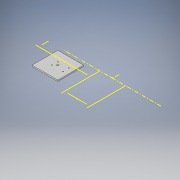
# Autodesk Inventor part: BT002_trajan20_21
Saved by Autodesk Inventor 2022.2 (Build 262287000, 287)
## iProperties
Company: HTBLA Kaindorf
RuleStatus: InUse
Created: 2022-06-07
Part Number: BT002_trajan20_21
Project: Zeichenmaschine_v2
Material: Generisch
Description: GM_Platte
Document SubType Name: Modeling
Designer: trajan20
Density: 1 g/cm^3
Appearance: Vorgabe
Mass: 25.3953 g
Surface Area: 141.888 cm^2
Volume: 25.3953 cm^3
AfterDocNew0: iProperties-Editor_aufrufen
Author: jan
Keywords: 2021
Autodesk Inventor part; units mm, degrees
ref_plane "YZ Plane" through (0, 0, 0) normal (1, 0, 0) x (0, 1, 0)
ref_plane "XZ Plane" through (0, 0, 0) normal (0, 1, 0) x (-1, 0, 0)
ref_plane "XY Plane" through (0, 0, 0) normal (0, 0, 1) x (1, 0, 0)
derived "MS000_trajan20_21_Zeichenmaschine_Inventor_Masterskizze.ipt"
sketch "Skizze19" plane through (30, -140, -50) normal (1, 0, 0) x (0, 1, 0)
  line L0 (10, -4) -> (-70, -4)
  line L1 (-70, -4) -> (-70, 0)
  line L2 (-70, 0) -> (10, 0)
  line L3 (10, 0) -> (10, -4)
  line L4 (-50, 10) -> (-10, 10)
  point P0 (140, 50)
  point P1 (-60, 0)
  point P2 (0, 0)
sketch "Basis" plane through (0, 0, 0) normal (0, 0, 1) x (1, 0, 0)
  line L0 (0, 150) -> (0, -150)
  line L1 (-19.8908, 0) -> (0.1065, 0)
  line L2 (0, -9.9039) -> (0, 9.9039)
  line L3 (30, -50) -> (30, -210)
  line L4 (0, -200) -> (20, -200)
  line L5 (0, -40) -> (120, -40)
  line L6 (0, 40) -> (120, 40)
  line L7 (110, -30) -> (110, 30)
  point P0 (0, 0)
  point P1 (110, 0)
sketch "Skizze20" plane through (30, -210, -54) normal (0, 0, 1) x (1, 0, 0)
  line L0 (0, 80) -> (0, 0)
  line L1 (0, 40) -> (-76.2792, 40) construction
  line L2 (-30, -72) -> (-30, 432) construction
  line L3 (-39.185, 86.341) -> (-39.185, 32.94) construction
  line L4 (-20.815, 77.6067) -> (-20.815, 18.0773) construction
  line L5 (-55.3723, 65.32) -> (-12.0627, 65.32) construction
  line L6 (-51.5852, 30.95) -> (-17.9084, 30.95) construction
  circle A0 centre (-30, 40) radius 3
  circle A1 centre (-20.815, 30.95) radius 1.35
  circle A2 centre (-39.185, 30.95) radius 1.35
  circle A3 centre (-39.185, 65.32) radius 1.35
  circle A4 centre (-20.815, 65.32) radius 1.35
  point P0 (-30, 210)
extrude "Extrusion3" add sketch "Skizze19" along normal blind 10 and the other way blind 30
mirror "Spiegeln1" about plane through (0, -170, -52) normal (-1, 0, 0)
extrude "Extrusion4" cut sketch "Skizze20" along normal through all
equation "\"d5\" = 0.5 * Alu_Prof"
equation "\"d6\" = 0.5 * Bas_Ver_Breite"
equation "\"Alu_Prof\" = 20"
equation "\"Bas_Ver_Breite\" = 60"
